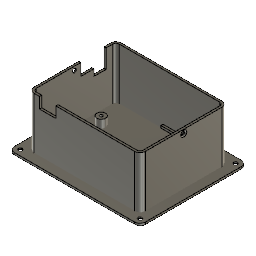
OUS-Box (Autodesk Fusion 360 design; units mm, degrees)
Autodesk Fusion 360 part; units mm, degrees
note: some values were not read from the file. Set by a fixed rule: which sketch regions a step uses; the direction of a hole.
sketch "Sketch1" plane through (0, 0, 0) normal (0, 0, 1) x (1, 0, 0)
  line L0 (60, -49) -> (-60, -49)
  line L1 (-60, -49) -> (-60, 49)
  line L2 (-60, 49) -> (60, 49)
  line L3 (60, 49) -> (60, -49)
  line L4 (60, -49) -> (-60, 49) construction
  line L5 (-60, -49) -> (60, 49) construction
  line L6 (-46, 38) -> (46, 38)
  line L7 (-49, 35) -> (-49, -35)
  arc A0 (-46, 38) -> (-49, 35) centre (-46, 35) ccw
  line L8 (-46, -38) -> (46, -38)
  arc A1 (-49, -35) -> (-46, -38) centre (-46, -35) ccw
  line L9 (49, 35) -> (49, -35)
  arc A2 (49, 35) -> (46, 38) centre (46, 35) ccw
  arc A3 (46, -38) -> (49, -35) centre (46, -35) ccw
  line L10 (-46, -40) -> (46, -40)
  arc A4 (46, -40) -> (51, -35) centre (46, -35) ccw
  line L11 (51, 35) -> (51, -35)
  arc A5 (51, 35) -> (46, 40) centre (46, 35) ccw
  line L12 (-46, 40) -> (46, 40)
  arc A6 (-46, 40) -> (-51, 35) centre (-46, 35) ccw
  line L13 (-51, 35) -> (-51, -35)
  arc A7 (-51, -35) -> (-46, -40) centre (-46, -35) ccw
  line L14 (10, 38) -> (10, 8) construction
  line L15 (-6, 38) -> (18.5, 38)
  line L16 (18.5, 38) -> (18.5, 36)
  line L17 (16.5, 36) -> (-6, 36)
  line L18 (-6, 36) -> (-6, 38)
  line L19 (18.5, 38) -> (20.5, 38)
  line L20 (20.5, 38) -> (20.5, 10)
  line L21 (20.5, 10) -> (18.5, 10)
  line L22 (18.5, 12) -> (18.5, 38)
  line L23 (18.5, 10) -> (10, 10)
  line L24 (10, 10) -> (10, 12)
  line L25 (10, 12) -> (18.5, 12)
  line L26 (10, 12) -> (18.5, 12)
  line L27 (16.5, 14) -> (10, 14)
  line L28 (10, 14) -> (10, 12)
  line L29 (16.5, 36) -> (16.5, 14)
  line L30 (18.5, 12) -> (18.5, 36)
  line L31 (-40, 15.5) -> (40, 15.5) construction
  line L32 (40, 15.5) -> (40, -20.5) construction
  line L33 (40, -20.5) -> (-40, -20.5) construction
  line L34 (-40, -20.5) -> (-40, 15.5) construction
  circle A8 centre (-54.75, 43.75) radius 1.75
  line L35 (0, 0) -> (-60, 0) construction
  line L36 (0, 0) -> (0, 49) construction
  circle A9 centre (-54.75, -43.75) radius 1.75
  circle A10 centre (54.75, 43.75) radius 1.75
  circle A11 centre (54.75, -43.75) radius 1.75
  line L37 (-32.5, 4.25) -> (32.5, 4.25)
  line L38 (32.5, 4.25) -> (32.5, -10.25)
  line L39 (32.5, -10.25) -> (-32.5, -10.25)
  line L40 (-32.5, -10.25) -> (-32.5, 4.25)
  line L41 (0, 0) -> (0, -49) construction
  circle A12 centre (0, -29.25) radius 6
  circle A13 centre (-37.5, 13) radius 1.35
  circle A14 centre (-37.5, 13) radius 4
  line L42 (-40, -2.5) -> (40, -2.5) construction
  circle A15 centre (-37.5, -18) radius 1.35
  circle A16 centre (-37.5, -18) radius 4
  circle A17 centre (37.5, 13) radius 1.35
  circle A18 centre (37.5, 13) radius 4
  circle A19 centre (37.5, -18) radius 1.35
  circle A20 centre (37.5, -18) radius 4
  dimension "d1" = 120
  dimension "d2" = 98
  dimension "d7" = 92
  dimension "d9" = 70
  dimension "d11" = 14
  dimension "d12" = 11
  dimension "d13" = 3
  dimension "d14" = 3
  dimension "d15" = 92
  dimension "d16" = 3
  dimension "d17" = 3
  dimension "d18" = 70
  dimension "d19" = 3
  dimension "d20" = 3
  dimension "d21" = 2
  dimension "d22" = 30
  dimension "d23" = 39
  dimension "d24" = 24.5
  dimension "d25" = 2
  dimension "d26" = 43
  dimension "d27" = 2
  dimension "d28" = 28
  dimension "d29" = 2
  dimension "d30" = 2
  dimension "d31" = 2
  dimension "d32" = 80
  dimension "d33" = 36
  dimension "d34" = 9
  dimension "d35" = 22.5
  dimension "d36" = 3.5
  dimension "d37" = 5.25
  dimension "d38" = 5.25
  dimension "d39" = 65
  dimension "d40" = 14.5
  dimension "d41" = 11.25
  dimension "d42" = 7.5
  dimension "d43" = 12
  dimension "d44" = 8.75
  dimension "d47" = 2.7
  dimension "d48" = 2.5
  dimension "d49" = 2.5
  dimension "d50" = 8
  dimension "d101" = 8.5
  constraint horizontal L0
  constraint perpendicular L0 L1
  constraint parallel L0 L2
  constraint parallel L1 L3
  constraint coincident L4 L35.start
  constraint coincident L5 L35.start
  constraint coincident L35.start L36.start
  constraint parallel L2 L6
  constraint parallel L1 L7
  constraint tangent L6 A0
  constraint horizontal L8
  constraint tangent L7 A1
  constraint tangent L8 A1
  constraint perpendicular L2 L9
  constraint tangent L6 A2
  constraint tangent L9 A3
  constraint coincident L6 L14.start
  constraint perpendicular L6 L14
  constraint horizontal L15
  constraint vertical L16
  constraint horizontal L17
  constraint vertical L18
  constraint coincident L6 L15.start
  constraint horizontal L19
  constraint vertical L20
  constraint horizontal L21
  constraint vertical L22
  constraint horizontal L23
  constraint vertical L24
  constraint horizontal L25
  constraint horizontal L26
  constraint horizontal L27
  constraint vertical L28
  constraint vertical L29
  constraint vertical L30
  constraint horizontal L31
  constraint vertical L32
  constraint horizontal L33
  constraint vertical L34
  constraint midpoint L1 L35.end
  constraint midpoint L2 L36.end
  constraint symmetric A8 L35 A9
  constraint symmetric A8 L36 A10
  constraint symmetric L36 A9 A11
  constraint horizontal L37
  constraint vertical L38
  constraint horizontal L39
  constraint vertical L40
  constraint midpoint L0 L41.end
  constraint coincident L41 A12.centre
  constraint concentric A13 A14
  constraint midpoint L34 L42.start
  constraint midpoint L32 L42.end
  constraint symmetric A13 L42 A15
  constraint symmetric A14 L42 A16
  constraint symmetric L41 A13 A17
  constraint symmetric L41 A14 A18
  constraint symmetric L41 A15 A19
  constraint symmetric L41 A16 A20
  measures "d1" distance of L1.end L2.end
  measures "d2" distance of L0.end L1.end
  measures "d7" distance of L6.start L6.end
  measures "d9" distance of L7.start L7.end
  measures "d11" horizontal distance of L1.end L6.start
  measures "d12" vertical distance of L1.end L6.start
  measures "d13" horizontal distance of L6.start L7.start
  measures "d14" vertical distance of L6.start L7.start
  measures "d15" distance of L8.start L8.end
  measures "d16" vertical distance of L7.end L8.start
  measures "d17" horizontal distance of L7.end L8.start
  measures "d18" distance of L9.start L9.end
  measures "d19" horizontal distance of L6.end L9.start
  measures "d20" vertical distance of L6.end L9.start
  measures "d22" distance of L14.start L14.end
  measures "d23" distance of L9 L14
  measures "d24" distance of L15.start L15.end
  measures "d25" distance of L15.start L17.end
  measures "d26" distance of L7.start L18
  measures "d27" distance of L15.end L19.end
  measures "d28" distance of L15.end L21.end
  measures "d29" distance of L21.end L22.start
  measures "d30" distance of L24.end L27.end
  measures "d31" distance of L16.end L17.start
  measures "d32" distance of L31.start L31.end
  measures "d33" distance of L31.start L33.end
  measures "d34" distance of L7 L34
  measures "d35" distance of L6 L31
  measures "d36" diameter of A8
  measures "d37" distance of L2 A8.centre
  measures "d38" distance of L1 A8.centre
  measures "d39" distance of L37.start L37.end
  measures "d40" distance of L37.start L39.end
  measures "d41" distance of L31 L37
  measures "d42" distance of L34 L40
  measures "d43" diameter of A12
  measures "d44" distance of L33 A12.centre
  measures "d47" diameter of A13
  measures "d48" distance of L34 A13.centre
  measures "d49" distance of L31 A13.centre
  measures "d50" diameter of A14
  measures "d101" distance of L24.end L22.start
extrude "Extrude1" add sketch "Sketch1" along normal blind 2 contours L0 L1 L2 L3 | L6 L7 A0 L8 A1 L9 A2 A3 L17 L18 L20 L21 L23 L24 L27 L28 L29 | L6 L15 L16 L17 L18 L22 L25 L26 L27 L28 L29 L30 | L6 L16 L19 L20 L21 L22 L23 L24 L25 L26 L30 | L10 A4 L11 A5 L12 A6 L13 A7 | A8 | A9 | A10 | A11 | A13 | A14 | A15 | A16 | A17 | A18 | A19 | A20 makes body 1
extrude "Extrude2" add sketch "Sketch1" along normal blind 5.5 separate body contours L6 L16 L19 L20 L21 L22 L23 L24 L25 L26 L30 makes body 2
extrude "Extrude3" add sketch "Sketch1" along normal blind 2 from surface at 3.5 contours L6 L15 L16 L17 L18 L22 L25 L26 L27 L28 L29 L30 bodies 2
extrude "Extrude4" add sketch "Sketch1" along normal blind 9 separate body contours A13 | A14 | A15 | A16 | A17 | A18 | A19 | A20 makes body 3 at (-33.505, -18.1994, 6) makes body 4 at (41.495, 12.8006, 6) makes body 5 at (-33.505, 12.8006, 6) makes body 6 at (41.495, -18.1994, 6)
extrude "Extrude5" cut sketch "Sketch1" along normal blind 4 from surface at 5 contours A13 | A15 | A17 | A19 bodies 3 4 5 6
extrude "Extrude6" add sketch "Sketch1" along normal blind 49 separate body contours L10 A4 L11 A5 L12 A6 L13 A7 makes body 7
fillet "Fillet1" radius 5 4 edges at (-60, -49, 1) (60, -49, 1) (60, 49, 1) (-60, 49, 1) on bodies 1
hole "Hole1" at (-54.75, -43.75, 0) at (-54.75, 43.75, 0) at (54.75, -43.75, 0) at (54.75, 43.75, 0) direction (0, 0, 1) diameter 3.5 depth 5 tip angle 118 countersink diameter 5.5 countersink angle 90 bodies 1
sketch "Sketch2" plane through (-51, 0, 0) normal (-1, 0, 0) x (0, -1, 0)
  line L0 (-35, 0) -> (35, 0)
  line L1 (35, 0) -> (35, 49)
  line L2 (35, 49) -> (-35, 49)
  line L3 (-35, 49) -> (-35, 0)
  line L4 (-40, 0) -> (-40, 49)
  line L5 (40, 0) -> (40, 49)
  line L6 (-29, 49) -> (-18, 49)
  line L7 (-18, 49) -> (-18, 32)
  line L8 (-18, 32) -> (-29, 32)
  line L9 (-29, 32) -> (-29, 49)
  line L10 (-18, 49) -> (-6, 49)
  line L11 (-6, 49) -> (-6, 38)
  line L12 (-6, 38) -> (-18, 38)
  line L13 (-18, 38) -> (-18, 49)
  line L14 (0, 0) -> (0, 49) construction
  circle A0 centre (0, 45.5) radius 1.75
  line L15 (35, 0) -> (-35, 0)
  line L16 (-35, 0) -> (-35, 49)
  line L17 (-35, 49) -> (35, 49)
  line L18 (35, 49) -> (35, 0)
  line L19 (0, 0) -> (0, 49) construction
  line L20 (-35, 0) -> (35, 0)
  line L21 (35, 0) -> (35, 49)
  line L22 (35, 49) -> (-35, 49)
  line L23 (-35, 49) -> (-35, 0)
  dimension "d72" = 11
  dimension "d73" = 17
  dimension "d74" = 11
  dimension "d75" = 12
  dimension "d76" = 11
  dimension "d77" = 3.5
  dimension "d78" = 3.5
  constraint horizontal L6
  constraint vertical L7
  constraint horizontal L8
  constraint vertical L9
  constraint coincident L2 L6.start
  constraint horizontal L10
  constraint vertical L11
  constraint horizontal L12
  constraint vertical L13
  constraint coincident L14.start L19.start
  constraint coincident L2 L14.end
  constraint perpendicular L2 L14
  constraint coincident L14 A0.centre
  measures "d72" distance of L6.start L6.end
  measures "d73" distance of L6.start L8.end
  measures "d74" distance of L4.end L9
  measures "d75" distance of L6.end L10.end
  measures "d76" distance of L6.end L12.end
  measures "d77" diameter of A0
  measures "d78" distance of L14.end A0.centre
extrude "Extrude7" cut sketch "Sketch2" against normal blind 2 contours L2 L6 L7 L8 L9 L13 L17 L22 | L2 L7 L10 L11 L12 L13 L17 L22 bodies 7
sketch "Sketch3" plane through (0, -40, 0) normal (0, -1, 0) x (1, 0, 0)
  line L0 (-46, 0) -> (46, 0)
  line L1 (46, 0) -> (46, 49)
  line L2 (46, 49) -> (-46, 49)
  line L3 (-46, 49) -> (-46, 0)
  line L4 (51, 0) -> (51, 49)
  line L5 (-51, 0) -> (-51, 49)
  line L6 (-41, 49) -> (-26, 49)
  line L7 (-26, 49) -> (-26, 39)
  line L8 (-26, 39) -> (-41, 39)
  line L9 (-41, 39) -> (-41, 49)
  dimension "d81" = 15
  dimension "d82" = 10
  dimension "d83" = 10
  constraint horizontal L6
  constraint vertical L7
  constraint horizontal L8
  constraint vertical L9
  constraint coincident L2 L6.start
  measures "d81" distance of L6.start L6.end
  measures "d82" distance of L6.start L8.end
  measures "d83" distance of L5.end L6.start
extrude "Extrude8" cut sketch "Sketch3" against normal blind 2 contours L2 L6 L7 L8 L9 bodies 7
sketch "Sketch4" plane through (51, 0, 0) normal (1, 0, 0) x (0, 1, 0)
  line L0 (-35, 0) -> (35, 0)
  line L1 (35, 0) -> (35, 49)
  line L2 (35, 49) -> (-35, 49)
  line L3 (-35, 49) -> (-35, 0)
  line L4 (0, 0) -> (0, 49) construction
  circle A0 centre (0, 45.5) radius 1.75
  dimension "d86" = 3.5
  dimension "d87" = 3.5
  constraint coincident L4.start origin
  constraint coincident L2 L4.end
  constraint perpendicular L2 L4
  constraint coincident L4 A0.centre
  measures "d86" diameter of A0
  measures "d87" distance of L4.end A0.centre
hole "Hole2" at (51, 0, 45.5) direction (-1, 0, 0) diameter 3.5 depth 5 tip angle 118 countersink diameter 5.5 countersink angle 90 bodies 7
hole "Hole3" at (-51, 0, 45.5) direction (1, 0, 0) diameter 3.5 depth 5 tip angle 118 countersink diameter 5.5 countersink angle 90 bodies 7
chamfer "Chamfer1" distance 1.7 angle 45 4 edges at (0, -10.25, 0) (-32.5, -3, 0) (0, 4.25, 0) (32.5, -3, 0) on bodies 1
sketch "Sketch5" plane through (0, 0, 49) normal (0, 0, 1) x (-1, 0, 0)
  line L0 (26, 38) -> (26, 40)
  line L1 (26, 40) -> (-46, 40)
  arc A0 (-46, 40) -> (-51, 35) centre (-46, 35) ccw
  line L2 (-51, 35) -> (-51, -35)
  arc A1 (-51, -35) -> (-46, -40) centre (-46, -35) ccw
  line L3 (-46, -40) -> (46, -40)
  arc A2 (46, -40) -> (51, -35) centre (46, -35) ccw
  line L4 (51, -35) -> (51, -29)
  line L5 (51, -29) -> (49, -29)
  line L6 (49, -29) -> (49, -35)
  arc A3 (46, -38) -> (49, -35) centre (46, -35) ccw
  line L7 (46, -38) -> (-46, -38)
  arc A4 (-49, -35) -> (-46, -38) centre (-46, -35) ccw
  line L8 (-49, -35) -> (-49, 35)
  arc A5 (-46, 38) -> (-49, 35) centre (-46, 35) ccw
  line L9 (-46, 38) -> (26, 38)
  line L10 (-52.5, 45) -> (52.5, 45)
  line L11 (52.5, 45) -> (52.5, -45)
  line L12 (52.5, -45) -> (-52.5, -45)
  line L13 (-52.5, -45) -> (-52.5, 45)
  line L14 (-52.5, 45) -> (52.5, -45) construction
  line L15 (52.5, 45) -> (-52.5, -45) construction
  dimension "d99" = 105
  dimension "d100" = 90
  constraint horizontal L10
  constraint perpendicular L10 L11
  constraint parallel L10 L12
  constraint parallel L11 L13
  constraint coincident L14 origin
  constraint coincident L15 origin
  measures "d99" distance of L11.end L12.end
  measures "d100" distance of L10.end L11.end
extrude "Extrude9" [suppressed]
equation "d11 = ( ( 120 - 92 ) / 2 ) * 1 mm"
equation "d28 = 25.5 mm + 2.5 mm"
equation "d35 = 27.5 mm - 5 mm"
equation "d44 = ( 17.5 / 2 ) * 1 mm"
